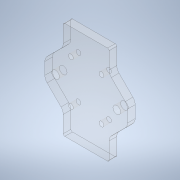
# Autodesk Inventor part: 103.010.01_Levilierebene_Stopper
Saved by Autodesk Inventor 2021 (Build 250183000, 183)
## iProperties
Created: 2021-11-23
Part Number: 103.010.01_Levilierebene_Stopper
Material: PMMA-Kunststoff
Document SubType Name: Modeling
Designer: Sebastian Seewald
Mass: 13.4802 g
Surface Area: 59.7659 cm^2
Volume: 11.347 cm^3
Density: 1.188 g/cm^3
Appearance: Polycarbonat - klar
Author: Sebastian Seewald
Autodesk Inventor part; units mm, degrees
ref_plane "YZ Plane" through (0, 0, 0) normal (1, 0, 0) x (0, 1, 0)
ref_plane "XZ Plane" through (0, 0, 0) normal (0, 1, 0) x (-1, 0, 0)
ref_plane "XY Plane" through (0, 0, 0) normal (0, 0, 1) x (1, 0, 0)
sketch "Skizze1" plane through (0, 0, 0) normal (0, 0, 1) x (1, 0, 0)
  line L0 (1, 0) -> (29, 0)
  line L1 (30, 1) -> (30, 63)
  line L2 (29, 64) -> (1, 64)
  line L3 (0, 63) -> (0, 1)
  arc A0 (0, 1) -> (1, 0) centre (1, 1) ccw
  arc A1 (29, 0) -> (30, 1) centre (29, 1) ccw
  arc A2 (30, 63) -> (29, 64) centre (29, 63) ccw
  arc A3 (1, 64) -> (0, 63) centre (1, 63) ccw
  line L4 (0, 50) -> (-12, 38)
  line L5 (-12, 38) -> (-12, 26)
  line L6 (-12, 26) -> (0, 14)
  line L7 (15, 64) -> (15, 0) construction
  line L8 (0, 32) -> (30, 32) construction
  circle A4 centre (-5, 32) radius 2.5
  circle A5 centre (5, 47) radius 1.6
  circle A6 centre (5, 19) radius 1.6
  line L9 (30, 50) -> (42, 38)
  line L10 (42, 38) -> (42, 26)
  line L11 (42, 26) -> (30, 14)
  circle A7 centre (35, 32) radius 2.5
  circle A8 centre (25, 47) radius 1.6
  circle A9 centre (25, 19) radius 1.6
  point P0 (0, 0)
  point P1 (30, 64)
  point P2 (30, 0)
  point P3 (0, 64)
  dimension "d31" = 64
  dimension "d32" = 30
  dimension "d33" = 1
  dimension "d34" = 12
  dimension "d36" = 45
  dimension "d37" = 45
  dimension "d38" = 12
  dimension "d39" = 5
  dimension "d40" = 7
  dimension "d41" = 6
  dimension "d42" = 3.2
  dimension "d43" = 3.2
  dimension "d44" = 19
  dimension "d45" = 28
  dimension "d46" = 10
  dimension "d48" = 40
  constraints: 24 end point, 10 centre point, 10 point on line, 8 point on circle, 8 symmetric about line, 8 tangent, 4 midpoint, 3 equal radius, 2 parallel, 1 horizontal, 1 perpendicular, 1 vertical, 1 vertical alignment, 3 other
  measures "d31" distance of point (30, 0) point (30, 64)
  measures "d32" distance of point (30, 64) point (0, 64)
  measures "d33" radius of A0
  measures "d34" distance of L4.end L5.end
  measures "d36" angle of L3 L4
  measures "d37" angle of L3 L6
  measures "d38" distance between parallel lines of L3 L5
  measures "d39" diameter of A4
  measures "d40" distance from line of L5 A4.centre
  measures "d41" vertical distance of L5.end A4.centre
  measures "d42" diameter of A5
  measures "d43" diameter of A6
  measures "d44" distance from line of A6.centre L0
  measures "d45" distance of A6.centre A5.centre
  measures "d46" distance from line of L7 A5.centre
  measures "d48" distance of A7.centre A4.centre
extrude "Extrusion1" add sketch "Skizze1" along normal blind 5
fillet "Rundung1" radius 5 8 edges at (0, 14, 2.5) (-12, 26, 2.5) (-12, 38, 2.5) (0, 50, 2.5) (30, 14, 2.5) (42, 26, 2.5) (42, 38, 2.5) (30, 50, 2.5)
